Autodesk Inventor part; units mm, degrees
(part 3 of 3)
sketch "Sketch53" plane through (0, 3, 0) normal (0, 1, 0) x (1, 0, 0)
  circle A0 centre (-21.9314, -99.0463) radius 1.5 projected
  circle A1 centre (-74.8109, -68.5163) radius 1.5 projected
  line L0 (-21.9314, -99.0463) -> (-74.8109, -68.5163)
  arc A2 (-95.9873, -38.0978) -> (-96.8317, -40.6032) centre (-94.9873, -39.8298) ccw projected
  line L1 (-96.9873, -39.8298) -> (-96.9873, 39.8298)
  arc A3 (-96.8317, 40.6032) -> (-95.9873, 38.0978) centre (-94.9873, 39.8298) ccw projected
  line L2 (-96.9873, 0) -> (-71.9873, 0)
  circle A4 centre (-72, 0) radius 1.5 projected
  line L3 (-95.9873, -38.0978) -> (-81, -29.4449) projected
  line L4 (-81, -29.4449) -> (-72, -24.2487)
  line L5 (-72, -24.2487) -> (-72, 0)
  line L6 (-72, 0) -> (-72, 24.249)
  line L7 (-81, 29.4449) -> (-95.9873, 38.0978) projected
  line L8 (-72, 24.249) -> (-81, 29.4449)
  arc A5 (-81, -29.4449) -> (-80, -27.7128) centre (-82, -27.7128) ccw projected
  line L9 (-81, 29.4449) -> (-81, -29.4449)
  point P0 (0, 0)
  dimension "d418" = 25
  dimension "d419" = 24.249
  constraints: 16 end point, 3 vertical, 2 point on circle, 1 collinear, 1 horizontal, 1 midpoint, 1 point on line
  measures "d418" distance of L2.start L2.end
  measures "d419" distance of L5.end L6.end
extrude "Extrusion43" cut sketch "Sketch53" against normal blind 3 contours L9 L2 A4 L5 L4 | L9 L8 L6 A4 L2 | A4 L2 L5 | A4 L6 L2
sketch "Sketch54" plane through (0, 3, 0) normal (0, 1, 0) x (1, 0, 0)
  arc A0 (-72, -1.5) -> (-72, 1.5) centre (-72, 0) ccw projected
  line L0 (-72, -1.5) -> (-69.8202, -1.5)
  line L1 (-69.8202, -1.5) -> (-69.8202, 1.5)
  line L2 (-69.8202, 1.5) -> (-72, 1.5)
  line L3 (-72, 1.5) -> (-72, -1.5)
  point P0 (0, 0)
  constraints: 8 end point, 2 parallel, 1 horizontal, 1 perpendicular
extrude "Extrusion44" add sketch "Sketch54" against normal blind 3
sketch "Sketch55" plane through (0, 3, 0) normal (0, 1, 0) x (1, 0, 0)
  line L0 (-72, 24.249) -> (-72, -24.2487) projected
  line L1 (-72, 0.0001) -> (-64, 0.0001)
  circle A0 centre (-64, 0.0001) radius 1.5
  point P0 (0, 0)
  dimension "d424" = 8
  dimension "d425" = 3
  constraints: 2 end point, 1 centre point, 1 coincident, 1 horizontal, 1 midpoint
  measures "d424" distance of L1.start L1.end
  measures "d425" diameter of A0
extrude "Extrusion45" cut sketch "Sketch55" against normal blind 3
sketch "Sketch56" plane through (0, 3, 0) normal (0, 1, 0) x (1, 0, 0)
  line L0 (-72, -24.2487) -> (-72, 24.249) projected
  line L1 (-81, 29.4449) -> (-72, 24.249) projected
  line L2 (-86.1476, 32.4167) -> (-77.1636, 27.23)
  line L3 (-77.1636, 27.23) -> (-76.0427, 29.1716)
  line L4 (-72, 24.249) -> (-81, 29.4449) projected
  line L5 (-76.0427, 29.1716) -> (-85.0267, 34.3582)
  line L6 (-85.0267, 34.3582) -> (-86.1476, 32.4167)
  point P0 (0, 0)
  constraints: 8 end point, 3 perpendicular, 2 point on line
extrude "Extrusion46" add sketch "Sketch56" against normal blind 3
sketch "Sketch57" plane through (0, 3, 0) normal (0, 1, 0) x (1, 0, 0)
  line L0 (-86.1475, 32.4168) -> (-95.9873, 38.0978) projected
  line L1 (-95.9873, 38.0978) -> (-84.9671, 31.7353)
  line L2 (-84.9671, 31.7353) -> (-84.0706, 33.2881)
  line L3 (-84.0706, 33.2881) -> (-95.0908, 39.6506)
  line L4 (-95.0908, 39.6506) -> (-95.9873, 38.0978)
  point P0 (0, 0)
  constraints: 8 end point, 3 perpendicular, 1 collinear
extrude "Extrusion47" add sketch "Sketch57" against normal blind 3
sketch "Sketch58" plane through (-86.1475, 0, -32.4168) normal (-0.8660374, 0, -0.4999792) x (-0.4999792, 0, 0.8660374)
  point P0 (-14.9978, 0)
sketch "Sketch59" plane through (0, 3, 0) normal (0, 1, 0) x (1, 0, 0)
  line L0 (-72, -24.2487) -> (-72, 24.249) projected
  line L1 (-86.1475, 32.4168) -> (-95.9873, 38.0978) projected
  line L2 (-72, 24.249) -> (-95.9873, 38.0978)
  line L3 (-95.9873, 38.0978) -> (-94.9667, 39.8655)
  line L4 (-94.9667, 39.8655) -> (-70.9794, 26.0167)
  line L5 (-70.9794, 26.0167) -> (-72, 24.249)
  point P0 (0, 0)
  constraints: 8 end point, 3 perpendicular
extrude "Extrusion48" add sketch "Sketch59" against normal blind 3
sketch "Sketch60" plane through (0, 3, 0) normal (0, 1, 0) x (1, 0, 0)
  line L0 (-72, 24.249) -> (-72, -24.2487) projected
  line L1 (-86.1475, 32.4168) -> (-95.9873, 38.0978) projected
  line L2 (-72, 24.249) -> (-95.9873, 38.0978)
  line L3 (-95.9873, 38.0978) -> (-94.8555, 40.0582)
  line L4 (-94.8555, 40.0582) -> (-70.8682, 26.2094)
  line L5 (-70.8682, 26.2094) -> (-72, 24.249)
  point P0 (0, 0)
  constraints: 8 end point, 3 perpendicular
extrude "Extrusion49" cut sketch "Sketch60" against normal blind 3
sketch "Sketch61" plane through (0, 3, 0) normal (0, 1, 0) x (1, 0, 0)
  line L0 (-70.8682, 26.2094) -> (-72, 24.249) projected
  line L1 (-71.4341, 25.2292) -> (-72.8511, 22.7748)
  line L2 (-72.8511, 22.7748) -> (-95.9873, 36.1322)
  line L3 (-95.9873, 36.1322) -> (-95.9873, 38.0978)
  line L4 (-95.9873, 38.0978) -> (-92.6118, 37.4559)
  line L5 (-92.6118, 37.4559) -> (-74.7348, 27.1348)
  line L6 (-72, 24.249) -> (-95.9873, 38.0978) projected
  line L7 (-74.7348, 27.1348) -> (-71.4341, 25.2292)
  point P0 (0, 0)
  constraints: 12 end point, 2 collinear, 1 midpoint, 1 parallel, 1 perpendicular, 1 vertical
extrude "Extrusion50" cut sketch "Sketch61" against normal blind 3
sketch "Sketch62" plane through (0, 3, 0) normal (0, 1, 0) x (1, 0, 0)
  line L0 (-94.8555, 40.0582) -> (-95.9873, 38.0978) projected
  line L1 (-72, 24.249) -> (-70.8682, 26.2094) projected
  line L2 (-95.9873, 38.0978) -> (-72, 24.249)
  line L3 (-70.8682, 26.2094) -> (-94.8555, 40.0582) projected
  line L4 (-72, 24.249) -> (-70.8682, 26.2094)
  point P0 (0, 0)
  constraints: 4 end point, 2 perpendicular
extrude "Extrusion51" add sketch "Sketch62" against normal blind 3
sketch "Sketch63" plane through (0, 3, 0) normal (0, 1, 0) x (1, 0, 0)
  circle A0 centre (0, 0) radius 105
  line L0 (-95.9873, -38.0978) -> (-72, -24.2487) projected
  line L1 (-94.2993, -37.1232) -> (-95.6387, -37.8965)
  line L2 (-95.6387, -37.8965) -> (-97.5, -38.9711)
  line L3 (-94.2993, -37.1232) -> (-72, -24.2487)
  circle A1 centre (-89.5067, -43.5938) radius 1.5 projected
  line L4 (-89.5067, -43.5938) -> (-93.5067, -36.6656)
  constraints: 8 end point, 4 point on line, 1 coincident, 1 collinear, 1 perpendicular, 3 other
fillet "Fillet21" radius 2 2 edges at (-72, 1.5, -24.249) (-72, 1.5, 24.2487)
sketch "Sketch64" plane through (0, 3, 0) normal (0, 1, 0) x (1, 0, 0)
  arc A0 (-95.9873, -38.0978) -> (-96.8317, -40.6032) centre (-94.9873, -39.8298) ccw projected
  line L0 (-96.9873, -39.8298) -> (-96.9873, 39.8298)
  arc A1 (-96.8317, 40.6032) -> (-95.9873, 38.0978) centre (-94.9873, 39.8298) ccw projected
  line L1 (-96.9873, 0) -> (-96.9873, -39.8298)
  line L2 (-96.9873, 0) -> (-67.9873, 0)
  line L3 (-95.9873, 38.0978) -> (-73, 24.8263) projected
  line L4 (-95.9873, 38.0978) -> (0, 0)
  line L5 (-95.9873, -38.0978) -> (0, 0)
  line L6 (-67.9873, 0) -> (-67.9873, -26.9845)
  line L7 (-67.9873, 0) -> (-67.9873, 26.9845)
  dimension "d443" = 29
  constraints: 14 end point, 3 point on line, 2 point on circle, 1 collinear, 1 horizontal, 1 midpoint, 1 parallel, 1 vertical
  measures "d443" distance of L1.start L2.end
extrude "Extrusion52" cut sketch "Sketch64" against normal blind 3 contours A0 L0 L2 L6 L5 | L0 A1 L4 L7 L2
sketch "Sketch65" plane through (0, 3, 0) normal (0, 1, 0) x (1, 0, 0)
  point P0 (0, 0)
  point P1 (-67.9873, -26.9845)
  point P2 (-67.9873, 26.9845)
fillet "Fillet22" radius 20 2 edges at (-67.9873, 1.5, 26.9845) (-67.9873, 1.5, -26.9845)
sketch "Sketch67" plane through (0, 3, 0) normal (0, 1, 0) x (1, 0, 0)
  line L0 (-83.8878, -56.804) -> (-74.5008, -55.8027)
  line L1 (-74.5008, -55.8027) -> (-58.1867, -48.7933)
  line L2 (-58.1867, -48.7933) -> (-54.5151, -37.2779)
  line L3 (-54.5151, -37.2779) -> (-64.6954, -27.4313)
  line L4 (-64.6954, -27.4313) -> (-72.2854, -30.6924)
  line L5 (-72.2854, -30.6924) -> (-81.9884, -34.8613)
  line L6 (-81.9884, -34.8613) -> (-87.9873, -41.0635)
  line L7 (-87.9873, -41.0635) -> (-85.1497, -44.9743)
  line L8 (-85.1497, -44.9743) -> (-88.8435, -48.7933)
  line L9 (-88.8435, -48.7933) -> (-83.8878, -56.804)
  point P0 (0, 0)
  constraints: 20 end point, 2 parallel, 1 perpendicular, 1 point on line
extrude "Extrusion53" add sketch "Sketch67" against normal blind 3
sketch "Sketch68" plane through (0, 3, 0) normal (0, 1, 0) x (1, 0, 0)
  point P0 (0, 0)
body "Solid1"
